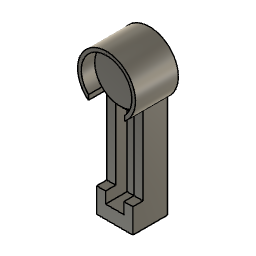
Haptic Sleeve Schematic v1 (Autodesk Fusion 360 archive; units mm, degrees)
design "Haptic sleeve angle motor mount"
Autodesk Fusion 360 part; units mm, degrees
sketch "Sketch1" plane through (0, 0, 0) normal (0, 0, 1) x (1, 0, 0)
  line L0 (3.6895, 0.0143) -> (-3.9305, 0.0143)
  line L1 (1.7795, -1.1857) -> (-2.0205, -1.1857)
  line L2 (-2.0205, 1.2143) -> (1.7795, 1.2143)
  line L3 (-2.0205, -1.1857) -> (-2.0205, 1.2143)
  line L4 (1.7795, 1.2143) -> (1.7795, -1.1857)
  line L5 (-2.0205, -1.1857) -> (1.7795, 1.2143) construction
  line L6 (1.7795, -1.1857) -> (-2.0205, 1.2143) construction
  line L7 (-3.8495, 4.0143) -> (-3.8495, 3.9643)
  line L8 (-3.9305, 3.9643) -> (-3.8805, 3.9643)
  line L9 (-3.8805, 3.9643) -> (3.6395, 3.9643)
  line L10 (3.6395, 3.9643) -> (3.6395, -1.1357)
  line L11 (3.6395, -1.1357) -> (-3.8805, -1.1357)
  line L12 (-3.8805, -1.1357) -> (-3.8805, 3.9643)
  point P0 (-0.1205, 0.0143)
  point P1 (-0.1205, 0.0143)
  dimension "d1" = 3.8
  dimension "d2" = 2.4
  dimension "d4" = 0.05
  dimension "d7" = 0.05
  constraint midpoint P0 L0
  constraint horizontal L1
  constraint perpendicular L1 L3
  constraint parallel L1 L2
  constraint parallel L3 L4
  constraint coincident P1 L6
  constraint coincident P1 L5
  constraint horizontal L9
  constraint vertical L10
  constraint horizontal L11
  constraint vertical L12
  measures "d1" distance of L2.start L2.end
  measures "d2" distance of L2.start L1.end
  measures "d4" distance of L7.start L7.end
  measures "d7" distance of L8.start L8.end
extrude "Extrude1" add sketch "Sketch1" along normal blind 12 contours L0 L4 L10 L11 | L0 L2 L3 L4 L9 L10 L12 | L0 L3 L11 L12
sketch "Sketch2" plane through (0, 0, 12) normal (0, 0, 1) x (-1, 0, 0)
  line L0 (2.0205, 1.1357) -> (2.0205, -1.2143)
  line L1 (2.0205, -1.2143) -> (-1.7795, -1.2143)
  line L2 (-1.7795, -1.2143) -> (-1.7795, 1.1357)
  line L3 (-1.7795, 1.1357) -> (-3.6395, 1.1357)
  line L4 (-3.6395, 1.1357) -> (-3.6395, -3.9643)
  line L5 (-3.6395, -3.9643) -> (3.8805, -3.9643)
  line L6 (3.8805, -3.9643) -> (3.8805, 1.1357)
  line L7 (3.8805, 1.1357) -> (2.0205, 1.1357)
  line L8 (3.8805, -3.9643) -> (-3.6395, -3.9643)
  line L9 (-3.6395, -3.9643) -> (-3.6395, 1.1357)
  line L10 (-3.6395, 1.1357) -> (3.8805, 1.1357)
  line L11 (3.8805, 1.1357) -> (3.8805, -3.9643)
  constraint horizontal L8
  constraint vertical L9
  constraint horizontal L10
  constraint vertical L11
  constraint coincident L3.end L4.start
  constraint coincident L5.end L6.start
extrude "Extrude2" add sketch "Sketch2" along normal blind 12
sketch "Sketch3" plane through (0, -1.1357, 0) normal (0, -1, 0) x (1, 0, 0)
  line L0 (1.7795, 0) -> (3.6395, 0)
  line L1 (3.6395, 0) -> (3.6395, 24)
  line L2 (3.6395, 24) -> (-3.8805, 24)
  line L3 (-3.8805, 24) -> (-3.8805, 0)
  line L4 (-3.8805, 0) -> (-2.0205, 0)
  line L5 (-2.0205, 0) -> (-2.0205, 12)
  line L6 (-2.0205, 12) -> (1.7795, 12)
  line L7 (1.7795, 12) -> (1.7795, 0)
  line L8 (-0.1205, 12) -> (-0.1205, 24)
  circle A0 centre (-0.1205, 18) radius 5.25
  circle A1 centre (-0.1205, 18) radius 6
  dimension "d12" = 10.5
  constraint midpoint L6 L8.start
  constraint midpoint L2 L8.end
  constraint midpoint L8 A0.centre
  constraint concentric A0 A1
  constraint coincident L8.end A1
  measures "d12" diameter of A0
extrude "Extrude3" add sketch "Sketch3" along normal blind 1 contours L1 L8 A0 A1 | L1 A0 A1 | L3 L8 A0 A1 | L1 L8 A0 | L1 A0 | L3 L8 A0 | L3 A0 A1 | L1 L8 A0 A1 | L3 L8 A0 A1 | L3 A0
extrude "Extrude4" add 2 faces at (-4.4308, -1.1357, 17.1359) (4.3641, -1.1357, 17.7033) along direction (0, 1, 0) blind 5.1
extrude "Extrude5" cut 2 faces at (3.4176, -1.1357, 23.2721) (-3.6585, -1.1357, 23.2721) along direction (0, 1, 0) blind 17
extrude "Extrude6" add sketch "Sketch3" along normal blind 4 contours L1 A0 A1 | L3 A0 A1 | L1 L8 A0 A1 | L3 L8 A0 A1 picked at (3.2445, 22.6489) picked at (-3.4854, 22.6489)
chamfer "Chamfer1" distance 0.75 angle 45 1 edges at (-0.1205, -2.1357, 12)
chamfer "Chamfer2" distance 0.25 angle 45 1 edges at (-0.1205, -1.3857, 12)
extrude "Extrude7" cut 1 faces at (-0.9635, -5.1357, 23.6766) along direction (0, 1, 0) blind 0.2
extrude "Extrude8" add 1 faces at (-0.7538, 3.0476, 0) along direction (0, 0, -1) blind 10
extrude "Extrude9" cut 1 faces at (-0.7538, 3.0476, -10) along direction (0, 0, 1) blind 2
sketch "Sketch4" plane through (0, -1.1357, 0) normal (0, -1, 0) x (1, 0, 0)
  line L0 (1.7795, -8) -> (3.6395, -8)
  line L1 (3.6395, -8) -> (3.6395, 13.3243)
  arc A0 (-0.1205, 12) -> (3.6395, 13.3243) centre (-0.1205, 18) ccw
  line L2 (-0.1205, 12) -> (1.7795, 12)
  line L3 (1.7795, 12) -> (1.7795, -8)
  line L4 (-3.8805, -8) -> (-2.0205, -8)
  line L5 (-2.0205, -8) -> (-2.0205, 12)
  line L6 (-2.0205, 12) -> (-0.1205, 12)
  arc A1 (-3.8805, 13.3243) -> (-0.1205, 12) centre (-0.1205, 18) ccw
  line L7 (-3.8805, 13.3243) -> (-3.8805, -8)
  line L8 (3.6395, -8) -> (-3.8805, -8)
  line L9 (-3.8805, -8) -> (-3.8805, -2.9)
  line L10 (-3.8805, -2.9) -> (3.6395, -2.9)
  line L11 (3.6395, -2.9) -> (3.6395, -8)
  dimension "d29" = 5.1
  constraint horizontal L8
  constraint vertical L9
  constraint horizontal L10
  constraint vertical L11
  constraint coincident L0.end L1.start
  measures "d29" distance of L0.end L10.end
extrude "Extrude10" add sketch "Sketch4" along normal blind 2.1 contours L0 L1 L3 L8 L10 L11 | L3 L5 L8 L10 | L4 L5 L7 L8 L9 L10
sketch "Sketch5" plane through (0, -3.2357, 0) normal (0, -1, 0) x (1, 0, 0)
  line L0 (3.6395, -2.9) -> (-3.8805, -2.9)
  line L1 (-3.8805, -2.9) -> (-3.8805, -8)
  line L2 (-3.8805, -8) -> (3.6395, -8)
  line L3 (3.6395, -8) -> (3.6395, -2.9)
  line L4 (-3.8805, -2.9) -> (-2.0205, -2.9)
  line L5 (-2.0205, -2.9) -> (-2.0205, 12)
  line L6 (-2.0205, 12) -> (-0.1205, 12)
  arc A0 (-3.8805, 13.3243) -> (-0.1205, 12) centre (-0.1205, 18) ccw
  line L7 (-3.8805, 13.3243) -> (-3.8805, -2.9)
  line L8 (1.7795, -2.9) -> (3.6395, -2.9)
  line L9 (3.6395, -2.9) -> (3.6395, 13.3243)
  arc A1 (-0.1205, 12) -> (3.6395, 13.3243) centre (-0.1205, 18) ccw
  line L10 (-0.1205, 12) -> (1.7795, 12)
  line L11 (1.7795, 12) -> (1.7795, -2.9)
  line L12 (-2.0205, -2.9) -> (1.7795, -2.9)
  line L13 (1.7795, -2.9) -> (1.7795, -5.25)
  line L14 (1.7795, -5.25) -> (-2.0205, -5.25)
  line L15 (-2.0205, -5.25) -> (-2.0205, -2.9)
  dimension "d32" = 2.35
  constraint horizontal L12
  constraint vertical L13
  constraint horizontal L14
  constraint vertical L15
  constraint coincident L4.end L5.start
  measures "d32" distance of L4.end L14.end
extrude "Extrude11" cut sketch "Sketch5" against normal blind 2.5 contours L0 L12 L13 L14 L15
extrude "Extrude12" add 1 faces at (0.5129, -1.1357, -7.0833) along direction (0, 1, 0) blind 2.5

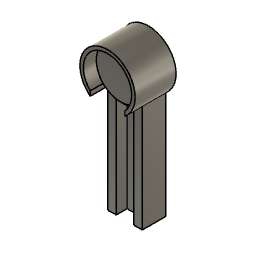
design "Haptic sleeve motor mount"
Autodesk Fusion 360 part; units mm, degrees
sketch "Sketch1" plane through (0, 0, 0) normal (0, 0, 1) x (1, 0, 0)
  line L0 (3.6895, 0.0143) -> (-3.9305, 0.0143)
  line L1 (1.7795, -1.1857) -> (-2.0205, -1.1857)
  line L2 (-2.0205, 1.2143) -> (1.7795, 1.2143)
  line L3 (-2.0205, -1.1857) -> (-2.0205, 1.2143)
  line L4 (1.7795, 1.2143) -> (1.7795, -1.1857)
  line L5 (-2.0205, -1.1857) -> (1.7795, 1.2143) construction
  line L6 (1.7795, -1.1857) -> (-2.0205, 1.2143) construction
  line L7 (-3.8495, 4.0143) -> (-3.8495, 3.9643)
  line L8 (-3.9305, 3.9643) -> (-3.8805, 3.9643)
  line L9 (-3.8805, 3.9643) -> (3.6395, 3.9643)
  line L10 (3.6395, 3.9643) -> (3.6395, -1.1357)
  line L11 (3.6395, -1.1357) -> (-3.8805, -1.1357)
  line L12 (-3.8805, -1.1357) -> (-3.8805, 3.9643)
  point P0 (-0.1205, 0.0143)
  point P1 (-0.1205, 0.0143)
  dimension "d1" = 3.8
  dimension "d2" = 2.4
  dimension "d4" = 0.05
  dimension "d7" = 0.05
  constraint midpoint P0 L0
  constraint horizontal L1
  constraint perpendicular L1 L3
  constraint parallel L1 L2
  constraint parallel L3 L4
  constraint coincident P1 L6
  constraint coincident P1 L5
  constraint horizontal L9
  constraint vertical L10
  constraint horizontal L11
  constraint vertical L12
  measures "d1" distance of L2.start L2.end
  measures "d2" distance of L2.start L1.end
  measures "d4" distance of L7.start L7.end
  measures "d7" distance of L8.start L8.end
extrude "Extrude1" add sketch "Sketch1" along normal blind 12 contours L0 L4 L10 L11 | L0 L2 L3 L4 L9 L10 L12 | L0 L3 L11 L12
sketch "Sketch2" plane through (0, 0, 12) normal (0, 0, 1) x (-1, 0, 0)
  line L0 (2.0205, 1.1357) -> (2.0205, -1.2143)
  line L1 (2.0205, -1.2143) -> (-1.7795, -1.2143)
  line L2 (-1.7795, -1.2143) -> (-1.7795, 1.1357)
  line L3 (-1.7795, 1.1357) -> (-3.6395, 1.1357)
  line L4 (-3.6395, 1.1357) -> (-3.6395, -3.9643)
  line L5 (-3.6395, -3.9643) -> (3.8805, -3.9643)
  line L6 (3.8805, -3.9643) -> (3.8805, 1.1357)
  line L7 (3.8805, 1.1357) -> (2.0205, 1.1357)
  line L8 (3.8805, -3.9643) -> (-3.6395, -3.9643)
  line L9 (-3.6395, -3.9643) -> (-3.6395, 1.1357)
  line L10 (-3.6395, 1.1357) -> (3.8805, 1.1357)
  line L11 (3.8805, 1.1357) -> (3.8805, -3.9643)
  constraint horizontal L8
  constraint vertical L9
  constraint horizontal L10
  constraint vertical L11
  constraint coincident L3.end L4.start
  constraint coincident L5.end L6.start
extrude "Extrude2" add sketch "Sketch2" along normal blind 12
sketch "Sketch3" plane through (0, -1.1357, 0) normal (0, -1, 0) x (1, 0, 0)
  line L0 (1.7795, 0) -> (3.6395, 0)
  line L1 (3.6395, 0) -> (3.6395, 24)
  line L2 (3.6395, 24) -> (-3.8805, 24)
  line L3 (-3.8805, 24) -> (-3.8805, 0)
  line L4 (-3.8805, 0) -> (-2.0205, 0)
  line L5 (-2.0205, 0) -> (-2.0205, 12)
  line L6 (-2.0205, 12) -> (1.7795, 12)
  line L7 (1.7795, 12) -> (1.7795, 0)
  line L8 (-0.1205, 12) -> (-0.1205, 24)
  circle A0 centre (-0.1205, 18) radius 5.25
  circle A1 centre (-0.1205, 18) radius 6
  dimension "d12" = 10.5
  constraint midpoint L6 L8.start
  constraint midpoint L2 L8.end
  constraint midpoint L8 A0.centre
  constraint concentric A0 A1
  constraint coincident L8.end A1
  measures "d12" diameter of A0
extrude "Extrude3" add sketch "Sketch3" along normal blind 1 contours L1 L8 A0 A1 | L1 A0 A1 | L3 L8 A0 A1 | L1 L8 A0 | L1 A0 | L3 L8 A0 | L3 A0 A1 | L1 L8 A0 A1 | L3 L8 A0 A1 | L3 A0
extrude "Extrude4" add 2 faces at (-4.4308, -1.1357, 17.1359) (4.3641, -1.1357, 17.7033) along direction (0, 1, 0) blind 5.1
extrude "Extrude5" cut 2 faces at (3.4176, -1.1357, 23.2721) (-3.6585, -1.1357, 23.2721) along direction (0, 1, 0) blind 17
extrude "Extrude6" add sketch "Sketch3" along normal blind 4 contours L1 A0 A1 | L3 A0 A1 | L1 L8 A0 A1 | L3 L8 A0 A1 picked at (3.2445, 22.6489) picked at (-3.4854, 22.6489)
chamfer "Chamfer1" distance 0.75 angle 45 1 edges at (-0.1205, -2.1357, 12)
chamfer "Chamfer2" distance 0.25 angle 45 1 edges at (-0.1205, -1.3857, 12)
extrude "Extrude7" cut 1 faces at (-0.9635, -5.1357, 23.6766) along direction (0, 1, 0) blind 0.2
extrude "Extrude8" add 1 faces at (-0.7538, 3.0476, 0) along direction (0, 0, -1) blind 10
